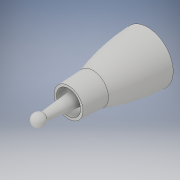
# Autodesk Inventor part: king
Saved by Autodesk Inventor 2019 (Build 230136000, 136)
## iProperties
Created: 2018-11-27
Part Number: king
Material: Generic
Document SubType Name: Modeling
Designer: Solomon Kritz
Density: 1 g/cm^3
Appearance: Default
Author: Solomon Kritz
Autodesk Inventor part; units mm, degrees
ref_plane "YZ Plane" through (0, 0, 0) normal (1, 0, 0) x (0, 1, 0)
ref_plane "XZ Plane" through (0, 0, 0) normal (0, 1, 0) x (-1, 0, 0)
ref_plane "XY Plane" through (0, 0, 0) normal (0, 0, 1) x (1, 0, 0)
sketch "Sketch2" plane through (0, 0, 0) normal (0, 1, 0) x (-1, 0, 0)
  line L0 (0, 0) -> (-10.5, 0)
  arc A0 (0, 47.5) -> (-1.5764, 43.0597) centre (0, 45) ccw
  line L1 (0, 45) -> (0, 47.5)
  line L2 (-1.5764, 43.0597) -> (-3.4552, 22.5826)
  line L3 (-3.4552, 22.5826) -> (-4.9552, 22.5826)
  line L4 (-4.9552, 22.5826) -> (-4.9552, 32.5826)
  line L5 (0, 45) -> (0, 0)
  arc A1 (-6.4552, 22.5826) -> (-10.5, 0) centre (71.2601, -2.9905) ccw
  line L6 (-4.9552, 32.5826) -> (-5.9552, 32.5826)
  line L7 (-5.9552, 32.5826) -> (-6.4552, 22.5826)
  dimension "d0" = 10.5
  dimension "d13" = 1.5
  dimension "d17" = 1
  constraints: 16 end point, 4 point on circle, 3 horizontal, 2 centre point, 2 vertical, 1 perpendicular, 1 point on line
  measures "d0" distance of L0.start L0.end
  measures "d13" distance of L2.end L3.end
  measures "d17" distance of L4.end L6.end
revolve "Revolution1" add sketch "Sketch2" angle 360 about axis through (0, 0, 45) along (0, 0, -1)
body "Solid1"
